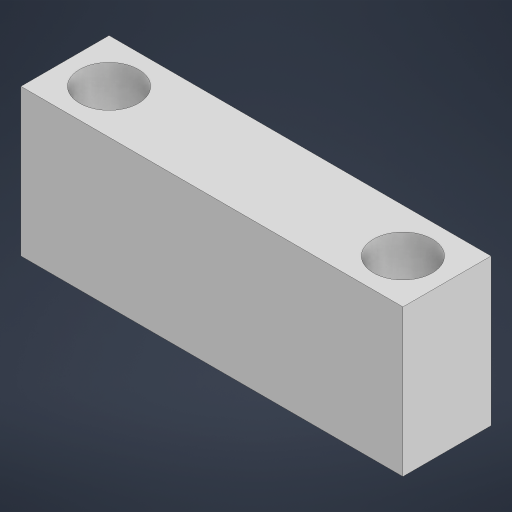
# Autodesk Inventor part: link
Saved by Autodesk Inventor 2024.3 (Build 283343000, 343)
## iProperties
Created: 2024-09-28
Part Number: link
Material: Generic
Document SubType Name: Modeling
Designer: sam
Density: 1 g/cm^3
Appearance: Default
Author: sam
Autodesk Inventor part; units mm, degrees
ref_plane "YZ Plane" through (0, 0, 0) normal (1, 0, 0) x (0, 1, 0)
ref_plane "XZ Plane" through (0, 0, 0) normal (0, 1, 0) x (-1, 0, 0)
ref_plane "XY Plane" through (0, 0, 0) normal (0, 0, 1) x (1, 0, 0)
sketch "Sketch1" plane through (0, 0, 0) normal (0, 1, 0) x (-1, 0, 0)
  line L0 (-6.5, -1.5) -> (6.5, -1.5)
  line L1 (6.5, 3.5) -> (6.5, 3.5)
  line L2 (6.5, 1.5) -> (-6.5, 1.5)
  line L3 (-6.5, 3.5) -> (-6.5, 3.5)
  line L4 (-6.5, -1.5) -> (6.5, 1.5) construction
  line L5 (6.5, -1.5) -> (-6.5, 1.5) construction
  circle A0 centre (5, 0) radius 1
  line L6 (-6.5, 1.5) -> (-6.5, -1.5)
  line L7 (6.5, 1.5) -> (6.5, -1.5)
  line L8 (-6.5, 1.5) -> (-7.5, 1.5)
  circle A1 centre (-5, 0) radius 1
  point P0 (0, 0)
  dimension "d0" = 3
  dimension "d1" = 13
  dimension "d3" = 2
  dimension "d6" = 1.5
  dimension "d8" = 1.5
  dimension "d21" = 2
  dimension "d22" = 1.5
  dimension "d23" = 1.5
  constraints: 18 end point, 4 point on line, 3 perpendicular, 2 centre point, 2 horizontal, 2 midpoint, 2 parallel
  measures "d0" distance of L2.start L0.end
  measures "d1" distance between parallel lines of L3 L1
  measures "d3" diameter of A0
  measures "d6" distance from line of L1 A0.centre
  measures "d8" distance from line of L2 A0.centre
  measures "d21" diameter of A1
  measures "d22" distance from line of L6 A1.centre
  measures "d23" distance from line of L2 A1.centre
extrude "Extrusion1" add sketch "Sketch1" along normal blind 5
body "Solid1"
